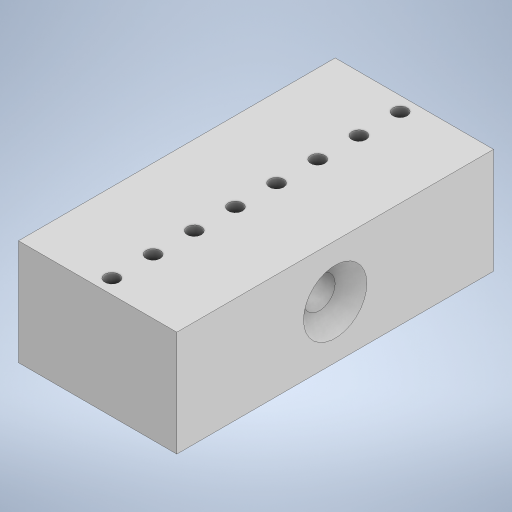
# Autodesk Inventor part: Prensa FO
Saved by Autodesk Inventor 2024.2 (Build 282272000, 272)
## iProperties
Created: 2026-02-17
Part Number: Prensa FO
Material: Generic
Document SubType Name: Modeling
Designer: ja.restrepo1
Density: 1 g/cm^3
Appearance: Default
Author: ja.restrepo1
Autodesk Inventor part; units mm, degrees
ref_plane "YZ Plane" through (0, 0, 0) normal (1, 0, 0) x (0, 1, 0)
ref_plane "XZ Plane" through (0, 0, 0) normal (0, 1, 0) x (-1, 0, 0)
ref_plane "XY Plane" through (0, 0, 0) normal (0, 0, 1) x (1, 0, 0)
sketch "Sketch1" plane through (0, 0, 0) normal (0, 1, 0) x (-1, 0, 0)
  line L0 (7.5, 15) -> (-7.5, 15)
  line L1 (-7.5, 15) -> (-7.5, -15)
  line L2 (-7.5, -15) -> (7.5, -15)
  line L3 (7.5, -15) -> (7.5, 15)
  circle A0 centre (0, 13.65) radius 0.675
  circle A1 centre (0, 9.75) radius 0.675
  circle A2 centre (0, 5.85) radius 0.675
  circle A3 centre (0, 1.95) radius 0.675
  circle A4 centre (0, -1.95) radius 0.675
  circle A5 centre (0, -5.85) radius 0.675
  circle A6 centre (0, -9.75) radius 0.675
  circle A7 centre (0, -13.65) radius 0.675
  point P0 (0, 0)
  point P1 (7.5, 0)
  point P2 (0, 15)
  dimension "d0" = 15
  dimension "d1" = 30
  dimension "d2" = 1.35
  dimension "d3" = 1.35
  dimension "d6" = 3.9
  dimension "d27" = 1.35
  constraints: 8 centre point, 8 end point, 2 midpoint, 2 parallel, 2 vertical alignment, 1 horizontal, 1 horizontal alignment, 1 perpendicular, 1 vertical, 14 other
  measures "d0" distance of L2.end L1.end
  measures "d1" distance of L1.end L0.end
  measures "d2" diameter of A0
  measures "d3" distance from line of L0 A0.centre
  measures "d6" distance of A0.centre A1.centre
  measures "d27" distance from line of L2 A7.centre
extrude "Cuerpo" add sketch "Sketch1" along normal mid plane 10
sketch "Sketch2" plane through (7.5, -5, -15) normal (1, 0, 0) x (0, 0, -1)
  point P0 (-15, 5)
  point P1 (-15, 5)
  constraints: 1 coincident
hole "BCAM3" at (7.5, 0, 0) direction (-1, 0, 0) diameter 3 depth 6 tip angle 118 countersink diameter 6 countersink angle 90
sketch "Sketch3" plane through (-7.5, -5, 15) normal (-1, 0, 0) x (0, 0, 1)
  circle A0 centre (-15, 5) radius 3 projected
  constraints: 1 coincident
hole "M3X0.6" at (-7.5, 0, 0) direction (1, 0, 0) diameter 2.459 end through all thread size "M3x0.5" class "6H" standard "ANSI Metric M Profile"
body "Solid1"
